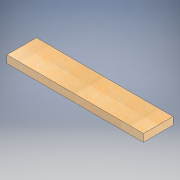
# Autodesk Inventor part: cap - 7
Saved by Autodesk Inventor 2022.2 (Build 262287010, 287A)
## iProperties
Created: 2022-03-21
Part Number: cap - 7
Material: Granite, Cut, Polished
Document SubType Name: Modeling
Designer: awelt
Mass: 196481 g
Surface Area: 18821.7 cm^2
Volume: 72770.9 cm^3
Density: 2.7 g/cm^3
Appearance: Amber Select
RuleStatus: InUse
AfterDocSave0: Convert in3 volume to ft3
Author: awelt
in3 to ft3: 2.57
Autodesk Inventor part; units mm, degrees
ref_plane "YZ Plane" through (0, 0, 0) normal (1, 0, 0) x (0, 1, 0)
ref_plane "XZ Plane" through (0, 0, 0) normal (0, 1, 0) x (-1, 0, 0)
ref_plane "XY Plane" through (0, 0, 0) normal (0, 0, 1) x (1, 0, 0)
sketch "Sketch1" plane through (0, 0, 0) normal (0, 1, 0) x (-1, 0, 0)
  line L0 (909.6375, -196.85) -> (-909.6375, -196.85)
  line L1 (-909.6375, -196.85) -> (-909.6375, 196.85)
  line L2 (-909.6375, 196.85) -> (909.6375, 196.85)
  line L3 (909.6375, 196.85) -> (909.6375, -196.85)
  line L4 (909.6375, -196.85) -> (-909.6375, 196.85) construction
  line L5 (-909.6375, -196.85) -> (909.6375, 196.85) construction
  point P0 (0, 0)
  dimension "d0" = 1819.275
  dimension "d1" = 393.7
  constraints: 12 end point, 2 midpoint, 2 parallel, 1 horizontal, 1 perpendicular
  measures "d0" distance of L1.end L2.end
  measures "d1" distance of L0.end L1.end
extrude "Extrusion1" add sketch "Sketch1" along normal blind 101.6
body "Solid1"
